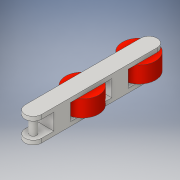
# Autodesk Inventor part: arm2
Saved by Autodesk Inventor 2016 (Build 200138000, 138)
## iProperties
Created: 2018-01-12
Part Number: arm2
Material: Generic
Document SubType Name: Modeling
Designer: New User
Density: 1 g/cm^3
Appearance: Default
Author: New User
Autodesk Inventor part; units mm, degrees
ref_plane "YZ Plane" through (0, 0, 0) normal (1, 0, 0) x (0, 1, 0)
ref_plane "XZ Plane" through (0, 0, 0) normal (0, 1, 0) x (-1, 0, 0)
ref_plane "XY Plane" through (0, 0, 0) normal (0, 0, 1) x (1, 0, 0)
sketch "Sketch1" plane through (0, 0, 0) normal (0, 1, 0) x (-1, 0, 0)
  line L0 (0, 0) -> (25.4, 0)
  line L1 (25.4, 0) -> (25.4, 203.2)
  line L2 (25.4, 203.2) -> (0, 203.2)
  line L3 (0, 203.2) -> (0, 0)
  dimension "d0" = 203.2
  dimension "d1" = 25.4
  constraints: 8 end point, 2 parallel, 1 horizontal, 1 perpendicular
  measures "d0" distance of L0.end L1.end
  measures "d1" distance of L0.start L0.end
extrude "Extrusion1" add sketch "Sketch1" along normal blind 38.1
sketch "Sketch2" plane through (0, 38.1, 0) normal (0, 1, 0) x (1, 0, 0)
  circle A0 centre (-12.7, -190.5) radius 5.2265
  line L0 (-25.4, 0) -> (-25.4, -203.2) projected
  line L1 (-25.4, -203.2) -> (0, -203.2) projected
  point P0 (0, 0)
  point P1 (-25.4, -12.7)
  point P2 (-25.4, -190.5)
  dimension "d5" = 10.453
  dimension "d6" = 12.7
  dimension "d7" = 12.7
  constraints: 1 centre point
  measures "d5" diameter of A0
  measures "d6" distance from line of L0 A0.centre
  measures "d7" distance from line of L1 A0.centre
sketch "Sketch3" plane through (0, 0, 203.2) normal (1, 0, 0) x (0, 0, -1)
  line L0 (0, 0) -> (0, 38.1) projected
  line L1 (0, 31.75) -> (31.75, 31.75)
  line L2 (31.75, 31.75) -> (31.75, 6.35)
  line L3 (31.75, 6.35) -> (0, 6.35)
  line L4 (0, 6.35) -> (0, 31.75)
  line L5 (0, 38.1) -> (203.2, 38.1) projected
  line L6 (57.15, 31.75) -> (120.65, 31.75)
  line L7 (120.65, 31.75) -> (120.65, 6.35)
  line L8 (120.65, 6.35) -> (57.15, 6.35)
  line L9 (57.15, 6.35) -> (57.15, 31.75)
  line L10 (146.05, 31.75) -> (209.55, 31.75)
  line L11 (209.55, 31.75) -> (209.55, 6.35)
  line L12 (209.55, 6.35) -> (146.05, 6.35)
  line L13 (146.05, 6.35) -> (146.05, 31.75)
  point P0 (203.2, 0)
  dimension "d8" = 25.4
  dimension "d9" = 6.35
  dimension "d10" = 203.2
  dimension "d11" = 31.75
  dimension "d16" = 63.5
  dimension "d17" = 63.5
  dimension "d18" = 25.4
  dimension "d19" = 25.4
  constraints: 24 end point, 6 parallel, 3 horizontal, 3 perpendicular, 3 point on line
  measures "d8" distance of L1.end L2.end
  measures "d9" distance between parallel lines of L5 L1
  measures "d10" distance of L0.end L5.end
  measures "d11" distance of L2.end L3.end
  measures "d16" distance of L6.start L6.end
  measures "d17" distance of L10.start L10.end
  measures "d18" distance between parallel lines of L9 L2
  measures "d19" distance between parallel lines of L13 L7
extrude "Extrusion4" cut sketch "Sketch3" against normal blind 68.2625
extrude "Extrusion3" add sketch "Sketch2" against normal blind 38.1
sketch "Sketch4" plane through (0, 6.35, 146.05) normal (0, 1, 0) x (1, 0, 0)
  circle A0 centre (-13.5299, 31.75) radius 25.4
  circle A1 centre (-15.1186, 120.65) radius 25.4
  line L0 (0, 63.5) -> (-25.4, 63.5) projected
  line L1 (0, 88.9) -> (-25.4, 88.9) projected
  point P0 (0, 146.05)
  dimension "d22" = 31.75
  dimension "d23" = 31.75
  dimension "d24" = 50.8
  constraints: 2 centre point, 1 equal radius
  measures "d22" distance from line of L0 A0.centre
  measures "d23" distance from line of L1 A1.centre
  measures "d24" diameter of A0
extrude "Extrusion5" add sketch "Sketch4" along normal blind 25.4
fillet "Fillet2" radius 12.7 8 edges at (0, 34.925, 0) (0, 3.175, 0) (-25.4, 3.175, 0) (-25.4, 34.925, 0) (0, 34.925, 203.2) (-25.4, 34.925, 203.2) (0, 3.175, 203.2) (-25.4, 3.175, 203.2)
body "Solid1"
